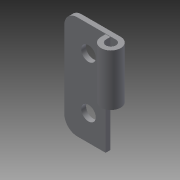
# Autodesk Inventor part: 2838_left
Saved by Autodesk Inventor 2014 SP2 (Build 180246200, 246)
## iProperties
Created: 2018-07-20
Part Number: 2838_left
Material: Generic
Catalog Web Link: www.cadenas.de
Description: 2830, 2831, 2832, 2833, 2835, 2836, 2837, 2838, 2839, 2840, 2841, 2842, 2830-Black, 2831-Black, 2832-Black, 2833-Black, 2835-Black, 2836-Black, 2837-Black, 2838-Black, 2839-Black, 2840-Black, 2841-Black, 2842-Black_left-Economy Lift-Off Hinges
Vendor: 8020
Document SubType Name: Modeling
Designer: psadmin
Manufacturer: 8020
Mass: 3.6839 g
Surface Area: 36.6433 cm^2
Volume: 3.6839 cm^3
Density: 1 g/cm^3
Appearance: PSOLRGB-191-191-191
Category: PARTsolutions
Company: 8020
Title: 2838_left
Author: Cadenas PARTsolutions
Comments: Economy Lift-Off Hinges
PSOL_IDENT_0: {$CADENAS_DATA\23d-libs\8020\inch\panels_and_doors\2830_left.prj},382 {VTYP=3D},{NB=2838_left},{LINA=
PSOL_IDENT_1: 2838_left},{NN=2830, 2831, 2832, 2833, 2835, 2836, 2837, 2838, 2839, 2840, 2841, 2842, 2830-Black, 2
PSOL_IDENT_2: 831-Black, 2832-Black, 2833-Black, 2835-Black, 2836-Black, 2837-Black, 2838-Black, 2839-Black, 2840-
PSOL_IDENT_3: Black, 2841-Black, 2842-Black_left},{DATE=16.03.2018 08:23:49},{GEOMDATE=20.11.2017 20:37:10},{VERSI
PSOL_IDENT_4: ON=},{LINEID=10},{WBVAR=TYPE,FINISH},{WBNUMERIC=}  {NB=2838_left},{LINA=2838_left},{KT=DUMMY},{PN=28
PSOL_IDENT_5: 38},{SERIES=10 Series},{TYPE=5},{MAT=Aluminum},{FINISH=CA},{A=2.000},{B=1.000},{C=1.000},{D=0.531},{
PSOL_IDENT_6: E=0.281},{F=0.500},{G=0.195},{H=0.187},{J=0.093},{K=0.062},{CAP=40},{R=0.381},{P=0.009},{NO=8},{CLR=
PSOL_IDENT_7: .75,.75,.75}
NN: 2830, 2831, 2832, 2833, 2835, 2836, 2837, 2838, 2839, 2840, 2841, 2842, 2830-Black, 2831-Black, 2832-Black, 2833-Black, 2835-Black, 2836-Black, 2837-Black, 2838-Black, 2839-Black, 2840-Black, 2841-Black, 2842-Black_left
NT: Economy Lift-Off Hinges
NB: 2838_left
NBSYN: $PN._left
LINA: 2838_left
PN: 2838
SERIES: 10 Series
TYPE: Right Hinge Long Pin
MAT: Aluminum
FINISH: Clear Anodize
A: 2
B: 1
C: 1
D: 0.531
E: 0.281
F: 0.5
G: 0.195
H: 0.187
J: 0.093
K: 0.062
CAP: 40
R: 0.381
SUPPLIER: 8020
ARTICLENO: 2838_left
BOMINFO: 2838_left
CREATOR: CADENAS GmbH
Autodesk Inventor part; units mm, degrees
sketch "Sketch_1" plane through (0, 0, 0) normal (0, 1, 0) x (-1, 0, 0)
  line L0 (25.4, 0) -> (25.4, 2.3622)
  line L1 (25.4, 2.3622) -> (0, 2.3622)
  arc A0 (2.4765, 4.8387) -> (0, 2.3622) centre (0, 4.8387) ccw
  line L2 (2.4765, 4.8387) -> (2.4765, 2.5527)
  line L3 (2.4765, 2.5527) -> (4.8387, 2.5527)
  line L4 (4.8387, 2.5527) -> (4.8387, 4.8387)
  arc A1 (4.8387, 4.8387) -> (0, 0) centre (0, 4.8387) ccw
  line L5 (0, 0) -> (25.4, 0)
  constraints: 12 end point, 4 point on circle, 2 centre point
extrude "Extrusion1" add sketch "Sketch_1" along normal mid plane 50.8
sketch "Sketch_3" plane through (0, 0, 0) normal (0, 0, 1) x (1, 0, 0)
  line L0 (-50.8, 50.8) -> (-50.8, -50.8)
  line L1 (-50.8, -50.8) -> (25.4, -50.8)
  line L2 (25.4, -50.8) -> (25.4, 50.8)
  line L3 (25.4, 50.8) -> (-50.8, 50.8)
  arc A0 (-25.4, -19.05) -> (-19.05, -25.4) centre (-19.05, -19.05) ccw
  line L4 (-19.05, -25.4) -> (-5.0673, -25.4)
  line L5 (-5.0673, -25.4) -> (-5.0673, 0.0254)
  line L6 (-5.0673, 0.0254) -> (12.7, 0.0254)
  line L7 (12.7, 0.0254) -> (12.7, 25.4)
  line L8 (12.7, 25.4) -> (-19.05, 25.4)
  arc A1 (-19.05, 25.4) -> (-25.4, 19.05) centre (-19.05, 19.05) ccw
  line L9 (-25.4, 19.05) -> (-25.4, -19.05)
  constraints: 20 end point, 4 point on circle, 2 centre point
extrude "Extrusion2" cut sketch "Sketch_3" along normal mid plane 25.4
sketch "Sketch_4" plane through (0, 0, 0) normal (0, 0, 1) x (1, 0, 0)
  circle A0 centre (-13.4874, 12.7) radius 3.5687
  constraints: 1 centre point
extrude "Extrusion3" cut sketch "Sketch_4" along normal mid plane 4.7244
sketch "Sketch_5" plane through (0, 0, 0) normal (0, 0, 1) x (1, 0, 0)
  circle A0 centre (-13.4874, -12.7) radius 3.5687
  constraints: 1 centre point
extrude "Extrusion4" cut sketch "Sketch_5" along normal mid plane 4.7244
ref_plane "to_dummy_XY" through (0, 0, 0) normal (0, -1, 0) x (1, 0, 0)
ref_plane "to_dummy_YZ" through (0, 0, 0) normal (1, 0, 0) x (0, 0, 1)
ref_plane "to_dummy_ZX" through (0, 0, 0) normal (0, 0, 1) x (0, -1, 0)
ref_plane "to_pin_XY" through (0, -25.4, 4.8387) normal (0, -1, 0) x (1, 0, 0)
ref_plane "to_pin_YZ" through (0, -25.4, 4.8387) normal (1, 0, 0) x (0, 0, 1)
ref_plane "to_pin_ZX" through (0, -25.4, 4.8387) normal (0, 0, 1) x (0, -1, 0)
ref_plane "to_right_XY" through (0, 0, 4.8387) normal (0, -1, 0) x (1, 0, 0)
ref_plane "to_right_YZ" through (0, 0, 4.8387) normal (1, 0, 0) x (0, 0, 1)
ref_plane "to_right_ZX" through (0, 0, 4.8387) normal (0, 0, 1) x (0, -1, 0)
body "Solid1"
